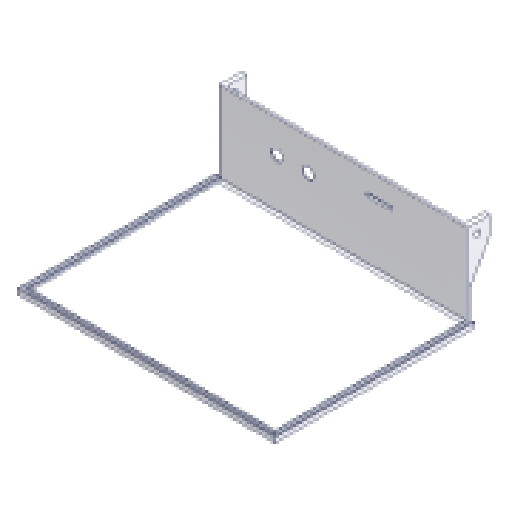
# Autodesk Inventor part: Tapa_chasis
Saved by Autodesk Inventor 2025 (Build 290162000, 162)
## iProperties
Created: 2026-02-01
Part Number: Tapa_chasis
Material: Plástico ABS
Document SubType Name: Modeling
Designer: HP
Density: 1.06 g/cm^3
Appearance: PTFE
Author: HP
Autodesk Inventor part; units mm, degrees
ref_plane "YZ Plane" through (0, 0, 0) normal (1, 0, 0) x (0, 1, 0)
ref_plane "XZ Plane" through (0, 0, 0) normal (0, 1, 0) x (-1, 0, 0)
ref_plane "XY Plane" through (0, 0, 0) normal (0, 0, 1) x (1, 0, 0)
sketch "Boceto1" plane through (0, 0, 0) normal (0, 1, 0) x (-1, 0, 0)
  line L0 (0, 0) -> (200, 0)
  line L1 (200, 0) -> (200, -156)
  line L2 (200, -156) -> (0, -156)
  line L3 (0, -156) -> (0, 0)
  dimension "d0" = 200
  dimension "d1" = 156
  constraints: 8 end point, 2 parallel, 1 horizontal, 1 perpendicular
  measures "d0" distance of L1.end L2.end
  measures "d1" distance of L0.end L1.end
extrude "Extrusión1" add sketch "Boceto1" along normal blind 2
sketch "Boceto2" plane through (0, 2, 0) normal (0, 1, 0) x (1, 0, 0)
  line L0 (0, 156) -> (-200, 156) projected
  line L1 (-200, 156) -> (-200, 0) projected
  line L2 (-200, 0) -> (0, 0) projected
  line L3 (0, 0) -> (0, 156) projected
  line L4 (3, 156) -> (3, -3)
  line L5 (3, -3) -> (-203, -3)
  line L6 (-203, -3) -> (-203, 156)
  line L7 (-200, 156) -> (-203, 156)
  line L8 (0, 156) -> (3, 156)
  line L9 (-200, 157) -> (-204, 157)
  line L10 (-204, 157) -> (-204, -4)
  line L11 (-204, -4) -> (4, -4)
  line L12 (4, -4) -> (4, 157)
  line L13 (4, 157) -> (0, 157)
  line L14 (-1, 155) -> (-199, 155)
  line L15 (-199, 155) -> (-199, 1)
  line L16 (-199, 1) -> (-1, 1)
  line L17 (-1, 1) -> (-1, 155)
  line L18 (-199, 155) -> (-200, 155)
  line L19 (-1, 155) -> (0, 155)
  line L20 (3, 156) -> (4, 156)
  line L21 (-203, 156) -> (-204, 156)
  dimension "d5" = 3
  dimension "d6" = 3
  dimension "d7" = 3
  dimension "d9" = 90
  dimension "d10" = 206
  dimension "d11" = 1
  dimension "d12" = 1
  constraints: 36 end point, 7 point on line, 2 perpendicular, 1 horizontal, 7 other
  measures "d5" distance of L0.start L4.start
  measures "d6" distance of L0.end L6.end
  measures "d7" distance between parallel lines of L2 L5
  measures "d9" angle of L4 L8
  measures "d10" distance between parallel lines of L4 L6
  measures "d11" distance between parallel lines of L6 L10
  measures "d12" distance between parallel lines of L3 L17
extrude "Extrusión2" add sketch "Boceto2" against normal blind 2 contours L8 L4 L5 L6 L7 L1 L2 L3 | L20 L12 L11 L10 L21 L6 L5 L4
extrude "Extrusión3" add sketch "Boceto2" along normal blind 2 contours L3 L2 L1 L18 L15 L16 L17 L19 | L20 L12 L11 L10 L21 L6 L5 L4
sketch "Boceto3" plane through (4, 0, -156) normal (0, 0, -1) x (-1, 0, 0)
  line L0 (0, 0) -> (208, 0) projected
  line L1 (208, 4) -> (208, 0) projected
  line L2 (207, 4) -> (208, 4) projected
  line L3 (207, 2) -> (207, 4) projected
  line L4 (1, 2) -> (207, 2) projected
  line L5 (1, 2) -> (1, 4) projected
  line L6 (0, 4) -> (1, 4) projected
  line L7 (0, 0) -> (0, 4) projected
  line L8 (5, 2) -> (4, 2) projected
  line L9 (5, 2) -> (5, 4) projected
  line L10 (4, 4) -> (5, 4) projected
  line L11 (4, 2) -> (4, 4) projected
  line L12 (204, 2) -> (203, 2) projected
  line L13 (204, 2) -> (204, 4) projected
  line L14 (203, 4) -> (204, 4) projected
  line L15 (203, 2) -> (203, 4) projected
  line L16 (204, 2) -> (4, 2)
  line L17 (4, 2) -> (4, 69)
  line L18 (4, 69) -> (204, 69)
  line L19 (204, 69) -> (204, 2)
  point P0 (4, 0)
  dimension "d17" = 200
  dimension "d18" = 67
  constraints: 8 end point, 2 parallel, 1 horizontal, 1 perpendicular
  measures "d17" distance of L17.end L18.end
  measures "d18" distance of L16.end L17.end
extrude "Extrusión4" add sketch "Boceto3" along normal mid plane 2
sketch "Boceto4" plane through (4, 0, -157) normal (0, 0, -1) x (-1, 0, 0)
  line L0 (207, 2) -> (1, 2) projected
  line L1 (207, 2) -> (207, 4) projected
  line L2 (1, 4) -> (207, 4) projected
  line L3 (1, 2) -> (1, 4) projected
  line L4 (204, 2) -> (204, 69) projected
  line L5 (204, 69) -> (4, 69) projected
  line L6 (4, 69) -> (4, 2) projected
  line L7 (4, 2) -> (1, 2) projected
  line L8 (1, 2) -> (1, 4) projected
  line L9 (1, 4) -> (0, 4) projected
  line L10 (0, 4) -> (0, 0) projected
  line L11 (0, 0) -> (208, 0) projected
  line L12 (208, 0) -> (208, 4) projected
  line L13 (208, 4) -> (207, 4) projected
  line L14 (207, 4) -> (207, 2) projected
  line L15 (207, 2) -> (204, 2) projected
  line L16 (204, 69) -> (200, 69)
  line L17 (200, 69) -> (200, 54)
  line L18 (200, 54) -> (204, 54)
  line L19 (204, 54) -> (204, 69)
  line L20 (4, 69) -> (204, 69) construction
  line L21 (104, 69) -> (104, 107.7155) construction
  line L22 (4, 69) -> (8, 69)
  line L23 (8, 69) -> (8, 54)
  line L24 (8, 54) -> (4, 54)
  line L25 (4, 54) -> (4, 69)
  point P0 (4, 0)
  point P1 (200, 69)
  dimension "d21" = 4
  dimension "d22" = 15
  constraints: 18 end point, 3 symmetric about line, 2 parallel, 1 horizontal, 1 midpoint, 1 perpendicular, 1 vertical
  measures "d21" distance of L18.end L17.end
  measures "d22" distance of L17.end L16.end
extrude "Extrusión5" add sketch "Boceto4" along normal blind 16 contours L18 L17 L5 L4 | L6 L5 L23 L24
sketch "Boceto8" plane through (0, 2, 0) normal (1, 0, 0) x (0, 0, -1)
  line L0 (157, 0) -> (0, 0) projected
  line L1 (157, 52) -> (157, 0) projected
  line L2 (157, 52) -> (173, 52) projected
  line L3 (173, 67) -> (173, 52) projected
  line L4 (155, 67) -> (173, 67) projected
  line L5 (155, 2) -> (155, 67) projected
  line L6 (0, 2) -> (155, 2) projected
  line L7 (0, 0) -> (0, 2) projected
  line L8 (173, 52) -> (157, 24.2872)
  line L9 (173, 52) -> (205, 52) construction
  point P0 (0, -2)
  dimension "d36" = 120
  constraints: 4 end point, 1 equal length, 1 horizontal, 1 point on line
  measures "d36" angle of L8 L9
extrude "Extrusión9" add sketch "Boceto8" against normal blind 4 contours L1 L2 L8
sketch "Boceto9" plane through (-200, 2, -157) normal (-1, 0, 0) x (0, 0, 1)
  line L0 (0, 67) -> (0, 24.2872) projected
  line L1 (0, 67) -> (-16, 67) projected
  line L2 (-16, 52) -> (-16, 67) projected
  line L3 (-16, 52) -> (0, 24.2872) projected
  line L4 (0, 52) -> (-16, 52) projected
  line L5 (-16, 52) -> (0, 52)
  point P0 (157, -2)
  constraints: 2 end point, 1 horizontal
extrude "Extrusión10" add sketch "Boceto9" against normal blind 4 contours L0 L3 L4
fillet "Empalme4" radius 3 2 edges at (-2, 26.2872, -157) (-198, 26.2872, -157)
fillet "Empalme5" radius 2 2 edges at (-198, 54, -173) (-2, 54, -173)
fillet "Empalme6" radius 2 1 edges at (-100, 0, -157)
fillet "Empalme7" radius 2 1 edges at (-100, 2, -155)
sketch "Boceto10" plane through (4, 0, -157) normal (0, 0, -1) x (-1, 0, 0)
  line L0 (204, 2) -> (4, 2) projected
  line L1 (204, 2) -> (204, 25.4833) projected
  line L2 (200, 25.4833) -> (204, 25.4833) projected
  line L3 (200, 25.4833) -> (200, 69) projected
  line L4 (200, 69) -> (8, 69) projected
  line L5 (8, 69) -> (8, 25.4833) projected
  line L6 (4, 25.4833) -> (8, 25.4833) projected
  line L7 (4, 25.4833) -> (4, 2) projected
  line L8 (170, 32.9273) -> (120, 32.9273)
  line L9 (120, 32.9273) -> (120, 52.9273)
  line L10 (120, 52.9273) -> (170, 52.9273)
  line L11 (170, 52.9273) -> (170, 32.9273)
  line L12 (120, 42.9273) -> (170, 42.9273) construction
  circle A0 centre (157.5, 42.9273) radius 4.65
  circle A1 centre (132.5, 42.9273) radius 4.65
  line L13 (65, 52.9273) -> (44.68, 52.9273)
  line L14 (44.68, 52.9273) -> (44.68, 50.3273)
  line L15 (44.68, 50.3273) -> (65, 50.3273)
  line L16 (65, 50.3273) -> (65, 52.9273)
  line L17 (65, 51.6273) -> (44.68, 51.6273) construction
  line L18 (65, 51.6273) -> (44.68, 51.6273) construction
  line L19 (65, 54.1273) -> (44.68, 54.1273)
  line L20 (44.68, 49.1273) -> (65, 49.1273)
  arc A2 (65, 49.1273) -> (65, 54.1273) centre (65, 51.6273) ccw
  arc A3 (44.68, 54.1273) -> (44.68, 49.1273) centre (44.68, 51.6273) ccw
  point P0 (4, 0)
  point P1 (54.84, 51.6273)
  dimension "d45" = 50
  dimension "d46" = 20
  dimension "d47" = 9.3
  dimension "d48" = 9.3
  dimension "d49" = 12.5
  dimension "d50" = 12.5
  dimension "d55" = 30
  dimension "d56" = 20.32
  dimension "d57" = 2.6
  dimension "d58" = 55
  dimension "d63" = 5
  constraints: 28 end point, 6 equal length, 5 midpoint, 4 centre point, 4 point on circle, 4 tangent, 3 point on line, 2 horizontal, 2 perpendicular
  measures "d45" distance of L9.end L10.end
  measures "d46" distance of L8.end L9.end
  measures "d47" diameter of A0
  measures "d48" diameter of A1
  measures "d49" distance from line of L11 A0.centre
  measures "d50" distance from line of L9 A1.centre
  measures "d55" distance between parallel lines of L3 L11
  measures "d56" distance of L15.end L14.end
  measures "d57" distance of L14.end L13.end
  measures "d58" distance between parallel lines of L9 L16
  measures "d63" diameter of A3
extrude "Extrusión11" cut sketch "Boceto10" against normal blind 1 contours L8 L9 L10 L11
extrude "Extrusión12" cut sketch "Boceto10" against normal through all contours A0 | A1
extrude "Extrusión13" cut sketch "Boceto10" against normal through all contours L16 L15 L14 L13 | A2 L20 A3 L19
sketch "Boceto11" plane through (-200, 4, -155) normal (-1, 0, 0) x (0, 0, 1)
  circle A0 centre (-8, 57) radius 2.5 projected
  point P0 (155, -4)
extrude "Extrusión14" cut sketch "Boceto11" against normal through all
sketch "Boceto5" plane through (4, 0, -157) normal (0, 0, -1) x (-1, 0, 0)
  line L0 (8, 68) -> (8, 50) projected
  line L1 (8, 50) -> (4, 50) projected
  line L2 (4, 50) -> (4, 2) projected
  line L3 (4, 2) -> (1, 2) projected
  line L4 (1, 2) -> (1, 4) projected
  line L5 (1, 4) -> (0, 4) projected
  line L6 (0, 4) -> (0, 0) projected
  line L7 (0, 0) -> (208, 0) projected
  line L8 (208, 0) -> (208, 4) projected
  line L9 (208, 4) -> (207, 4) projected
  line L10 (207, 4) -> (207, 2) projected
  line L11 (207, 2) -> (204, 2) projected
  line L12 (204, 2) -> (204, 50) projected
  line L13 (204, 50) -> (200, 50) projected
  line L14 (200, 50) -> (200, 68) projected
  line L15 (200, 68) -> (8, 68) projected
  line L16 (1, 4) -> (4, 4)
  line L17 (1, 4) -> (207, 4) projected
  line L18 (204, 4) -> (207, 4)
  point P0 (4, 0)
  constraints: 4 end point, 4 point on line, 1 collinear
sketch "Boceto6" plane through (0, 4, -156) normal (1, 0, 0) x (0, 0, -1)
  line L0 (0, 0) -> (2, 0) projected
  line L1 (2, 46) -> (2, 0) projected
  line L2 (2, 46) -> (20, 46) projected
  line L3 (20, 64) -> (20, 46) projected
  line L4 (0, 64) -> (20, 64) projected
  line L5 (0, 64) -> (0, 0) projected
  line L6 (2, 46) -> (20, 46) projected
  line L7 (2, 14.8231) -> (20, 46)
  line L8 (2, 14.8231) -> (38, 14.8231) construction
  point P0 (-156, -4)
  point P1 (1, 0)
  dimension "d27" = 60
  constraints: 4 end point, 1 equal length, 1 horizontal, 1 midpoint, 1 point on line
  measures "d27" angle of L8 L7
sketch "Boceto7" plane through (-200, 4, -156) normal (-1, 0, 0) x (0, 0, 1)
  line L0 (-1, 64) -> (-1, 46) projected
  line L1 (-1, 64) -> (-19, 64) projected
  line L2 (-19, 46) -> (-19, 64) projected
  line L3 (-2, 46) -> (-19, 46) projected
  line L4 (-19, 46) -> (-2, 46)
  line L5 (-1, 46) -> (-19, 46) projected
  point P0 (156, -4)
  constraints: 2 end point, 1 horizontal, 1 other
